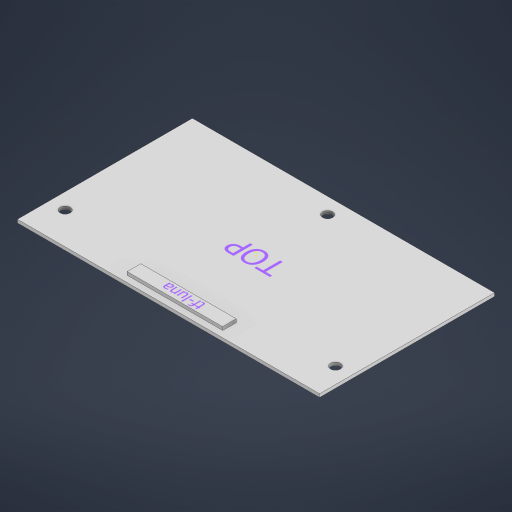
# Autodesk Inventor part: pcb
Saved by Autodesk Inventor 2024 (Build 280153000, 153)
## iProperties
Created: 2024-02-07
Part Number: pcb
Material: Všeobecné
Document SubType Name: Modeling
Designer: Simak
Density: 1 g/cm^3
Appearance: Výchozí
Author: Simak
Autodesk Inventor part; units mm, degrees
ref_plane "YZ Plane" through (0, 0, 0) normal (1, 0, 0) x (0, 1, 0)
ref_plane "XZ Plane" through (0, 0, 0) normal (0, 1, 0) x (-1, 0, 0)
ref_plane "XY Plane" through (0, 0, 0) normal (0, 0, 1) x (1, 0, 0)
sketch "Náčrt1" plane through (0, 0, 0) normal (0, 1, 0) x (-1, 0, 0)
  line L0 (-47.5, 27.5) -> (47.5, 27.5)
  line L1 (47.5, 27.5) -> (47.5, -27.5)
  line L2 (47.5, -27.5) -> (-47.5, -27.5)
  line L3 (-47.5, -27.5) -> (-47.5, 27.5)
  circle A0 centre (-42.5, 17.5) radius 1.6
  line L4 (-47.5, -27.5) -> (0, 0) construction
  line L5 (0, 0) -> (47.5, 27.5) construction
  line L6 (0, 0) -> (47.5, -27.5) construction
  circle A1 centre (42.5, 17.5) radius 1.6
  circle A2 centre (0, -22.5) radius 1.6
  dimension "d0" = 95
  dimension "d1" = 55
  dimension "d2" = 10
  dimension "d3" = 5
  dimension "d4" = 5
  dimension "d5" = 3.2
  dimension "d6" = 5
  constraints: 14 end point, 3 centre point, 2 equal length, 2 equal radius, 2 parallel, 1 horizontal, 1 horizontal alignment, 1 perpendicular, 1 vertical alignment
  measures "d0" distance of L0.start L0.end
  measures "d1" distance of L0.end L1.end
  measures "d2" distance from line of L0 A0.centre
  measures "d3" distance from line of L3 A0.centre
  measures "d4" distance from line of A1.centre L1
  measures "d5" diameter of A0
  measures "d6" distance from line of L2 A2.centre
extrude "Vysunutí1" add sketch "Náčrt1" along normal blind 1
sketch "Náčrt4" plane through (0, 1, 0) normal (0, 1, 0) x (1, 0, 0)
  line L0 (7.8805, -3.6441) -> (-7.5821, -3.6441) construction
  line L1 (-7.5821, -3.6441) -> (-7.5821, 2.7129) construction
  line L2 (-7.5821, 2.7129) -> (7.8805, 2.7129) construction
  line L3 (7.8805, 2.7129) -> (7.8805, -3.6441) construction
  point P0 (0, 0)
  constraints: 2 other
sketch "Náčrt2" plane through (0, 1, 0) normal (0, 1, 0) x (1, 0, 0)
  line L0 (15, -25.5) -> (-15, -25.5)
  line L1 (-15, -25.5) -> (-15, -21.2)
  line L2 (-15, -21.2) -> (15, -21.2)
  line L3 (15, -21.2) -> (15, -25.5)
  line L4 (15, -21.2) -> (0, -23.35) construction
  line L5 (0, -23.35) -> (-15, -21.2) construction
  line L6 (0, -23.35) -> (-15, -25.5) construction
  line L7 (-47.5, -27.5) -> (47.5, -27.5) projected
  point P0 (0, 0)
  dimension "d9" = 4.3
  dimension "d10" = 30
  dimension "d11" = 2
  constraints: 14 end point, 5 equal length, 1 horizontal, 1 perpendicular, 1 vertical alignment
  measures "d9" distance of L0.end L1.end
  measures "d10" distance of L1.end L2.end
  measures "d11" distance between parallel lines of L7 L0
extrude "Vysunutí2" add sketch "Náčrt2" along normal blind 1
sketch "Náčrt3" plane through (0, 2, 0) normal (0, 1, 0) x (1, 0, 0)
  line L0 (6.4228, -25.0535) -> (-10.4314, -25.0535) construction
  line L1 (-10.4314, -25.0535) -> (-10.4314, -21.2271) construction
  line L2 (-10.4314, -21.2271) -> (6.4228, -21.2271) construction
  line L3 (6.4228, -21.2271) -> (6.4228, -25.0535) construction
  point P0 (0, 0)
  constraints: 2 other
equation "\"d4\" = d3"
equation "\"d6\" = d3"
